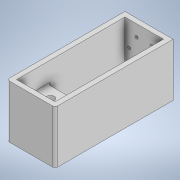
# Autodesk Inventor part: Link3_v2
Saved by Autodesk Inventor 2022 (Build 260153000, 153)
## iProperties
Created: 2022-06-10
Part Number: Link3_v2
Material: Generic
Document SubType Name: Modeling
Designer: Asus
Density: 1 g/cm^3
Appearance: Default
Author: Asus
Autodesk Inventor part; units mm, degrees
ref_plane "YZ Plane" through (0, 0, 0) normal (1, 0, 0) x (0, 1, 0)
ref_plane "XZ Plane" through (0, 0, 0) normal (0, 1, 0) x (-1, 0, 0)
ref_plane "XY Plane" through (0, 0, 0) normal (0, 0, 1) x (1, 0, 0)
sketch "Sketch1" plane through (0, 0, 0) normal (0, 1, 0) x (-1, 0, 0)
  line L0 (25, 22.5) -> (-25, 22.5)
  line L1 (-25, 22.5) -> (-25, -100)
  line L2 (-25, -100) -> (25, -100)
  line L3 (25, -100) -> (25, 22.5)
  circle A0 centre (0, 0) radius 4
  dimension "d0" = 50
  dimension "d1" = 22.5
  dimension "d2" = 25
  dimension "d3" = 122.5
  dimension "d4" = 8
  constraints: 8 end point, 2 parallel, 1 centre point, 1 coincident, 1 horizontal, 1 perpendicular
  measures "d0" distance between parallel lines of L3 L1
  measures "d1" distance from line of L0 point (0, 0)
  measures "d2" distance from line of L3 point (0, 0)
  measures "d3" distance of L0.end L1.end
  measures "d4" diameter of A0
extrude "Extrusion1" add sketch "Sketch1" along normal blind 5
sketch "Sketch2" plane through (0, 5, 0) normal (0, 1, 0) x (1, 0, 0)
  line L0 (-25, 100) -> (-25, -22.5) projected
  line L1 (25, -22.5) -> (25, 100) projected
  line L2 (-25, -22.5) -> (25, -22.5)
  line L3 (25, -22.5) -> (25, 100)
  line L4 (25, 100) -> (-25, 100)
  line L5 (-25, 100) -> (-25, -22.5)
  line L6 (-20, -17.5) -> (20, -17.5)
  line L7 (20, -17.5) -> (20, 95)
  line L8 (20, 95) -> (-20, 95)
  line L9 (-20, 95) -> (-20, -17.5)
  point P0 (0, 0)
  dimension "d7" = 5
  dimension "d8" = 5
  dimension "d9" = 5
  dimension "d10" = 5
  constraints: 16 end point, 4 parallel, 2 horizontal, 2 perpendicular
  measures "d7" distance between parallel lines of L8 L4
  measures "d8" distance between parallel lines of L7 L1
  measures "d9" distance between parallel lines of L2 L6
  measures "d10" distance between parallel lines of L0 L9
extrude "Extrusion2" add sketch "Sketch2" along normal blind 50
sketch "Sketch3" plane through (0, 5, 0) normal (0, 1, 0) x (1, 0, 0)
  line L0 (-20, 95) -> (-20, -17.5) projected
  line L1 (20, -17.5) -> (20, 95) projected
  line L2 (-20, -17.5) -> (20, -17.5)
  line L3 (20, -17.5) -> (20, 14.5)
  line L4 (20, 14.5) -> (-20, 14.5)
  line L5 (-20, 14.5) -> (-20, -17.5)
  point P0 (0, 0)
  dimension "d13" = 32
  constraints: 8 end point, 2 parallel, 1 horizontal, 1 perpendicular, 1 point on line
  measures "d13" distance between parallel lines of L2 L4
extrude "Extrusion3" add sketch "Sketch3" along normal blind 30
sketch "Sketch4" plane through (25, 0, -100) normal (0, 0, -1) x (-1, 0, 0)
  circle A0 centre (25, 22.5) radius 6.5
  line L0 (0, 0) -> (50, 0) projected
  line L1 (50, 0) -> (50, 55) projected
  circle A1 centre (25, 29.5) radius 15.5
  line L2 (25, 29.5) -> (45.4383, 29.5)
  line L3 (45.4383, 29.5) -> (2.3057, 29.5)
  line L4 (25, 29.5) -> (33.9734, 13.9576)
  line L5 (25, 29.5) -> (15.8246, 13.6078)
  line L6 (25, 29.5) -> (33.427, 44.096)
  line L7 (25, 29.5) -> (15.5571, 45.8556)
  circle A2 centre (40.5, 29.5) radius 1.5
  circle A3 centre (32.75, 42.9234) radius 1.5
  circle A4 centre (17.25, 42.9234) radius 1.5
  circle A5 centre (9.5, 29.5) radius 1.5
  circle A6 centre (17.25, 16.0766) radius 1.5
  circle A7 centre (32.75, 16.0766) radius 1.5
  point P0 (25, 0)
  dimension "d16" = 22.5
  dimension "d17" = 13
  dimension "d18" = 25
  dimension "d19" = 7
  dimension "d20" = 31
  dimension "d21" = 60
  dimension "d22" = 60
  dimension "d23" = 60
  dimension "d24" = 60
  dimension "d25" = 25
  dimension "d26" = 3
  dimension "d27" = 3
  dimension "d28" = 3
  dimension "d29" = 3
  dimension "d30" = 3
  dimension "d31" = 3
  constraints: 12 end point, 8 centre point, 7 point on line, 6 point on circle, 1 horizontal
  measures "d16" distance from line of L0 A0.centre
  measures "d17" diameter of A0
  measures "d18" distance from line of L1 A0.centre
  measures "d19" distance of L2.start A0.centre
  measures "d20" diameter of A1
  measures "d21" angle of L4 L5
  measures "d22" angle of L2 L4
  measures "d23" angle of L2 L6
  measures "d24" angle of L7 L6
  measures "d25" distance from line of L1 L2.start
  measures "d26" diameter of A3
  measures "d27" diameter of A2
  measures "d28" diameter of A4
  measures "d29" diameter of A5
  measures "d30" diameter of A6
  measures "d31" diameter of A7
extrude "Extrusion4" cut sketch "Sketch4" against normal blind 30 contours A0 L4 | L4 A0 L5 | L5 A0 | A7 A1 L4 | L4 A1 A7 | A2 A1 L2 | L2 A1 A2 | A5 A1 L3 | L3 A1 A5 | A3 A1 L6 | L6 A1 A3 | A4 A1 L7 | L7 A1 A4 | A6 A1 L5 | L5 A1 A6 | L4 A7 A1 | A1 A7 L4 | L2 A2 A1 | A1 A2 L2 | L3 A5 A1 | A1 A5 L3 | A1 A3 | L7 A4 A1 | A1 A4 L7 | L5 A6 A1 | A1 A6 L5 picked at (24.9025, 21.8029)
sketch "Sketch5" plane through (0, 0, 0) normal (0, -1, 0) x (1, 0, 0)
  circle A0 centre (0, 0) radius 4 projected
  circle A1 centre (0, 0) radius 9.5
  dimension "d34" = 19
  constraints: 1 centre point, 1 coincident
  measures "d34" diameter of A1
extrude "Extrusion5" cut sketch "Sketch5" against normal blind 12.5 contours A0 | A1
sketch "Sketch6" plane through (0, 0, 0) normal (0, -1, 0) x (1, 0, 0)
  circle A0 centre (0, 0) radius 9.5 projected
  circle A1 centre (0, 0) radius 11.5
  dimension "d37" = 23
  constraints: 1 centre point, 1 coincident
  measures "d37" diameter of A1
extrude "Extrusion6" cut sketch "Sketch6" against normal blind 6.5 contours A0 | A1
sketch "Sketch7" plane through (0, 12.5, 0) normal (0, -1, 0) x (1, 0, 0)
  circle A0 centre (0, 0) radius 9.5 projected
  circle A1 centre (0, 0) radius 6.2
  line L0 (0, 0) -> (0, 7.2993)
  line L1 (0, 0) -> (-6.3974, -3.6935)
  line L2 (0, 0) -> (6.4992, -3.7523)
  circle A2 centre (5.3694, -3.1) radius 1.45
  circle A3 centre (-5.3694, -3.1) radius 1.45
  circle A4 centre (0, 6.2) radius 1.45
  dimension "d40" = 12.4
  dimension "d41" = 120
  dimension "d42" = 120
  dimension "d43" = 2.9
  dimension "d44" = 2.9
  dimension "d45" = 2.9
  constraints: 6 end point, 4 centre point, 3 point on circle, 3 point on line, 1 coincident, 1 vertical
  measures "d40" diameter of A1
  measures "d41" angle of L1 L0
  measures "d42" angle of L2 L1
  measures "d43" diameter of A2
  measures "d44" diameter of A3
  measures "d45" diameter of A4
extrude "Extrusion7" cut sketch "Sketch7" against normal blind 30 contours A4 L0 A1 | A1 A4 | A2 A1 | A1 L2 A2 | L0 A4 A1 | A1 A2 L2 | A3 L1 A1 | A1 A3 | A3 A1 L1
fillet "Fillet1" radius 3 4 edges at (20, 20, -14.5) (-20, 20, -14.5) (25, 27.5, 22.5) (-25, 27.5, 22.5)
sketch "Sketch8" plane through (0, 35, 0) normal (0, 1, 0) x (1, 0, 0)
  circle A0 centre (-5.3694, 3.1) radius 1.45 projected
  circle A1 centre (-5.3694, 3.1) radius 4
  circle A2 centre (5.3694, 3.1) radius 1.45 projected
  circle A3 centre (5.3694, 3.1) radius 4
  circle A4 centre (0, -6.2) radius 1.45 projected
  circle A5 centre (0, -6.2) radius 4
  point P0 (0, 0)
  dimension "d49" = 8
  dimension "d50" = 8
  dimension "d51" = 8
  constraints: 3 centre point, 3 coincident
  measures "d49" diameter of A5
  measures "d50" diameter of A3
  measures "d51" diameter of A1
extrude "Extrusion8" cut sketch "Sketch8" against normal blind 7
body "Solid1"
